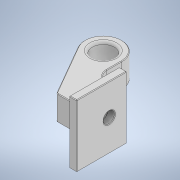
# Autodesk Inventor part: Fridge Hinge
Saved by Autodesk Inventor 2021 (Build 250183000, 183)
## iProperties
Created: 2020-12-04
Part Number: Fridge Hinge
Material: Generic
Document SubType Name: Modeling
Designer: ppxsp1
Density: 1 g/cm^3
Appearance: Default
Author: ppxsp1
Autodesk Inventor part; units mm, degrees
ref_plane "YZ Plane" through (0, 0, 0) normal (1, 0, 0) x (0, 1, 0)
ref_plane "XZ Plane" through (0, 0, 0) normal (0, 1, 0) x (-1, 0, 0)
sketch "Sketch4" plane through (0, 0, 0) normal (0, 1, 0) x (-1, 0, 0)
  circle A0 centre (0, 0) radius 4.375
  arc A1 (-7.375, 0) -> (6.3869, 3.6875) centre (0, 0) ccw
  line L0 (0, 0) -> (17, 0) construction
  line L1 (-7.375, 0) -> (-7.375, 6)
  line L2 (-11.375, 10) -> (-16.375, 10)
  line L3 (-16.375, 10) -> (-16.375, 24.0598)
  line L4 (6.3869, 3.6875) -> (-5.375, 24.0598)
  line L5 (6.3869, 3.6875) -> (29.9108, 3.6875) construction
  line L6 (-5.375, 24.0598) -> (-16.375, 24.0598)
  arc A2 (-7.375, 6) -> (-11.375, 10) centre (-11.375, 6) ccw
  point P0 (-7.375, 10)
  dimension "d18" = 8.75
  dimension "d19" = 7.375
  dimension "d23" = 9
  dimension "d25" = 120
  dimension "d27" = 11
  dimension "d29" = 10
  dimension "d30" = 4
  constraints: 14 end point, 4 horizontal, 4 point on circle, 4 tangent, 3 centre point, 3 point on line, 2 coincident, 1 equal length, 1 perpendicular, 1 vertical
  measures "d18" diameter of A0
  measures "d19" radius of A1
  measures "d23" distance of point (-7.375, 10) L2.end
  measures "d25" angle of L5 L4
  measures "d27" distance from line of L3 L4.end
  measures "d29" distance from line of L2 point (0, 0)
  measures "d30" radius of A2
extrude "Extrusion3" add sketch "Sketch4" along normal mid plane 10
sketch "Sketch5" plane through (16.375, -5, 10) normal (1, 0, 0) x (0, 0, -1)
  line L0 (0, 17.5) -> (-20, 17.5)
  line L1 (-20, 17.5) -> (-20, -7.5)
  line L2 (-20, -7.5) -> (0, -7.5)
  line L3 (0, -7.5) -> (0, 17.5)
  line L4 (0, 17.5) -> (-20, -7.5) construction
  line L5 (-20, 17.5) -> (0, -7.5) construction
  line L6 (0, 0) -> (0, 10) construction
  point P0 (10, 5)
  point P1 (-10, 5)
  point P2 (0, 5)
  point P3 (-10, 5)
  dimension "d35" = 20
  dimension "d36" = 25
  constraints: 12 end point, 4 midpoint, 2 parallel, 1 collinear, 1 horizontal, 1 horizontal alignment, 1 perpendicular
  measures "d35" distance of L2.end L1.end
  measures "d36" distance of L1.end L0.end
extrude "Extrusion4" add sketch "Sketch5" along normal blind 3
sketch "Sketch6" plane through (19.375, -5, 10) normal (1, 0, 0) x (0, 0, -1)
  line L0 (-14.0598, 0) -> (-14.0598, 10) projected
  line L1 (-14.0598, 10) -> (0, 10) projected
  line L2 (0, 0) -> (-14.0598, 0) projected
  line L3 (0, 0) -> (0, 10) projected
  circle A0 centre (-7, 5) radius 2.25
  point P0 (10, 5)
  dimension "d39" = 7
  dimension "d40" = 5
  dimension "d41" = 5
  dimension "d42" = 4.5
  constraints: 1 centre point
  measures "d39" distance from line of L3 A0.centre
  measures "d40" distance from line of L2 A0.centre
  measures "d41" distance from line of L1 A0.centre
  measures "d42" diameter of A0
extrude "Extrusion5" cut sketch "Sketch6" against normal up to next contours A0
ref_plane "Work Plane1" through (-2.375, -5, 10) normal (-1, 0, 0) x (0, 0, 1)
sketch "Sketch7" plane through (-2.375, -5, 10) normal (-1, 0, 0) x (0, 0, 1)
  circle A0 centre (7, 5) radius 2.25 projected
  circle A1 centre (7, 5) radius 4.25
  point P0 (-10, 5)
  dimension "d46" = 8.5
  constraints: 1 centre point, 1 coincident
  measures "d46" diameter of A1
extrude "Extrusion6" cut sketch "Sketch7" against normal up to surface (18.75 mm away)
fillet "Fillet1" radius 3 3 edges at (16.375, -5, 17.0299) (16.375, 0, 24.0598) (16.375, 5, 17.0299)
fillet "Fillet2" radius 1 3 edges at (5.375, 0, 24.0598) (4.375, -5, 0) (4.375, 5, 0)
chamfer "Chamfer1" distance 0.25 angle 45 35 edges at (16.375, 0, 19.25) (9.6637, -5, 24.0598) (5.4524, -5, 23.9258) (-0.6503, -5, 13.6236) (-1.9088, -5, -7.1237) (7.375, -5, 3) (8.5466, -5, 8.8284) (12.375, -5, 10) (15.4963, -5.8787, 10) (16.375, -10.25, 10) (15.4963, -5.8787, 24.9385) (-0.6503, 5, 13.6236) (5.4524, 5, 23.9258) (9.6637, 5, 24.0598) (15.4963, 5.8787, 24.9385) (-1.9088, 5, -7.1237) (7.375, 5, 3) (8.5466, 5, 8.8284) (12.375, 5, 10) (15.4963, 5.8787, 10) (16.375, 10.25, 10) (16.375, 0, 12.75) (19.375, 0, 10) (19.375, 0, 30) (16.375, 0, 30) (17.875, -12.5, 30) (19.375, -12.5, 20) (17.875, -12.5, 10) (16.375, -12.5, 20) (17.875, 12.5, 10) (19.375, 12.5, 20) (17.875, 12.5, 30) (16.375, 12.5, 20) (19.375, 0, 19.25) (-1.1547, 0, 12.75)
equation "\"d40\" = d41"
body "Solid3"
